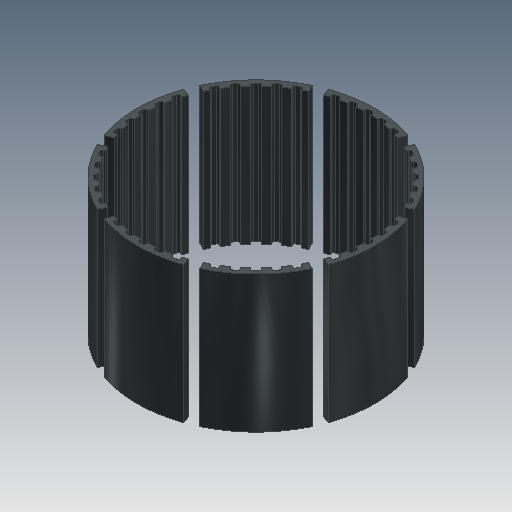
# Autodesk Inventor part: Nema 17 Stator Face
Saved by Autodesk Inventor 2020.2 (Build 242310000, 310)
## iProperties
Created: 2020-01-21
Part Number: Nema 17 Stator Face
Material: Iron, Ductile
Document SubType Name: Modeling
Designer: james
Density: 7.15 g/cm^3
Appearance: Iron Gray
Mass: 5.84467 g
Surface Area: 31.3117 cm^2
Volume: 0.817437 cm^3
Author: james
Autodesk Inventor part; units mm, degrees
ref_plane "YZ Plane" through (0, 0, 0) normal (1, 0, 0) x (0, 1, 0)
ref_plane "XZ Plane" through (0, 0, 0) normal (0, 1, 0) x (-1, 0, 0)
ref_plane "XY Plane" through (0, 0, 0) normal (0, 0, 1) x (1, 0, 0)
sketch "Sketch11" plane through (0, 0, 0) normal (0, 1, 0) x (-1, 0, 0)
  arc A0 (-4.3395, -12.2543) -> (4.3395, -12.2543) centre (0, 0) ccw
  arc A1 (-4.6399, -13.1027) -> (4.6399, -13.1027) centre (0, 0) ccw
  line L0 (4.6399, -13.1027) -> (4.3395, -12.2543)
  line L1 (-4.3395, -12.2543) -> (-4.6399, -13.1027)
  line L2 (4.3395, -12.2543) -> (0, 0) construction
  line L3 (0, 0) -> (-4.3395, -12.2543) construction
  arc A2 (5.5966, -11.7336) -> (11.7336, -5.5966) centre (0, 0) ccw
  arc A3 (5.9841, -12.5459) -> (12.5459, -5.9841) centre (0, 0) ccw
  line L4 (12.5459, -5.9841) -> (11.7336, -5.5966)
  line L5 (5.5966, -11.7336) -> (5.9841, -12.5459)
  line L6 (11.7336, -5.5966) -> (0, 0) construction
  line L7 (0, 0) -> (5.5966, -11.7336) construction
  arc A4 (12.2543, -4.3395) -> (12.2543, 4.3395) centre (0, 0) ccw
  arc A5 (13.1027, -4.6399) -> (13.1027, 4.6399) centre (0, 0) ccw
  line L8 (13.1027, 4.6399) -> (12.2543, 4.3395)
  line L9 (12.2543, -4.3395) -> (13.1027, -4.6399)
  line L10 (12.2543, 4.3395) -> (0, 0) construction
  line L11 (0, 0) -> (12.2543, -4.3395) construction
  arc A6 (11.7336, 5.5966) -> (5.5966, 11.7336) centre (0, 0) ccw
  arc A7 (12.5459, 5.9841) -> (5.9841, 12.5459) centre (0, 0) ccw
  line L12 (5.9841, 12.5459) -> (5.5966, 11.7336)
  line L13 (11.7336, 5.5966) -> (12.5459, 5.9841)
  line L14 (5.5966, 11.7336) -> (0, 0) construction
  line L15 (0, 0) -> (11.7336, 5.5966) construction
  arc A8 (4.3395, 12.2543) -> (-4.3395, 12.2543) centre (0, 0) ccw
  arc A9 (4.6399, 13.1027) -> (-4.6399, 13.1027) centre (0, 0) ccw
  line L16 (-4.6399, 13.1027) -> (-4.3395, 12.2543)
  line L17 (4.3395, 12.2543) -> (4.6399, 13.1027)
  line L18 (-4.3395, 12.2543) -> (0, 0) construction
  line L19 (0, 0) -> (4.3395, 12.2543) construction
  arc A10 (-5.5966, 11.7336) -> (-11.7336, 5.5966) centre (0, 0) ccw
  arc A11 (-5.9841, 12.5459) -> (-12.5459, 5.9841) centre (0, 0) ccw
  line L20 (-12.5459, 5.9841) -> (-11.7336, 5.5966)
  line L21 (-5.5966, 11.7336) -> (-5.9841, 12.5459)
  line L22 (-11.7336, 5.5966) -> (0, 0) construction
  line L23 (0, 0) -> (-5.5966, 11.7336) construction
  arc A12 (-12.2543, 4.3395) -> (-12.2543, -4.3395) centre (0, 0) ccw
  arc A13 (-13.1027, 4.6399) -> (-13.1027, -4.6399) centre (0, 0) ccw
  line L24 (-13.1027, -4.6399) -> (-12.2543, -4.3395)
  line L25 (-12.2543, 4.3395) -> (-13.1027, 4.6399)
  line L26 (-12.2543, -4.3395) -> (0, 0) construction
  line L27 (0, 0) -> (-12.2543, 4.3395) construction
  arc A14 (-11.7336, -5.5966) -> (-5.5966, -11.7336) centre (0, 0) ccw
  arc A15 (-12.5459, -5.9841) -> (-5.9841, -12.5459) centre (0, 0) ccw
  line L28 (-5.9841, -12.5459) -> (-5.5966, -11.7336)
  line L29 (-11.7336, -5.5966) -> (-12.5459, -5.9841)
  line L30 (-5.5966, -11.7336) -> (0, 0) construction
  line L31 (0, 0) -> (-11.7336, -5.5966) construction
  point P0 (0, -13)
  point P1 (9.1924, -9.1924)
  point P2 (13, 0)
  point P3 (9.1924, 9.1924)
  point P4 (0, 13)
  point P5 (-9.1924, 9.1924)
  point P6 (-13, 0)
  point P7 (-9.1924, -9.1924)
  dimension "d82" = 13
  dimension "d83" = 13.9
  dimension "d86" = 360
  dimension "d92" = 39
  constraints: 64 end point, 33 point on circle, 16 centre point, 8 concentric, 2 collinear, 1 coincident, 1 vertical alignment, 105 other
  measures "d82" radius of A0
  measures "d83" radius of A1
  measures "d92" angle of L1 L0
extrude "Extrusion7" add sketch "Sketch11" along normal mid plane 16
sketch "Sketch12" plane through (0, 8, 0) normal (0, 1, 0) x (1, 0, 0)
  line L0 (4.3395, 12.2543) -> (4.6399, 13.1027) projected
  line L1 (-4.6399, 13.1027) -> (-4.3395, 12.2543) projected
  arc A0 (0.45, 13.4425) -> (-0.45, 13.4425) centre (0, 0) ccw
  arc A1 (4.3395, 12.2543) -> (-4.3395, 12.2543) centre (0, 0) ccw
  line L2 (-0.45, 13.4425) -> (0, 0)
  line L3 (0, 0) -> (0.45, 13.4425)
  line L4 (0, 13.45) -> (0, 0) construction
  arc A2 (4.6399, 13.1027) -> (-4.6399, 13.1027) centre (0, 0) ccw construction
  arc A3 (4.4897, 12.6785) -> (-4.4897, 12.6785) centre (0, 0) ccw construction
  arc A4 (4.3395, 12.2543) -> (-4.3395, 12.2543) centre (0, 0) ccw construction
  point P0 (-0.4349, 12.9927)
  point P1 (0.4349, 12.9927)
  dimension "d91" = 39
  dimension "d94" = 0.9
  constraints: 7 point on circle, 6 end point, 3 centre point, 3 concentric, 2 midpoint, 1 coincident, 1 line through centre, 1 vertical
  measures "d91" angle of L0 L1
  measures "d94" distance of L3.end L2.start
extrude "Extrusion8" cut sketch "Sketch12" against normal blind 16 contours L3 A1 L2 A0
pattern_circular "Circular Pattern1" count 5 over 30 about axis through (0, 0, 0) along (0, 1, 0) of "Extrusion8" both ways yes
fillet "Fillet8" radius 0.25 10 edges at (-3.9138, 0, -12.868) (-3.0445, 0, -13.1009) (-2.2007, 0, -13.2687) (-1.3084, 0, -13.3862) (-0.45, 0, -13.4425) (0.45, 0, -13.4425) (1.3084, 0, -13.3862) (2.2007, 0, -13.2687) (3.0445, 0, -13.1009) (3.9138, 0, -12.868)
pattern_circular "Circular Pattern2" count 8 over 360 about axis through (0, 0, 0) along (0, 1, 0) of "Extrusion8", "Circular Pattern1", "Fillet8"
body "Solid6"
